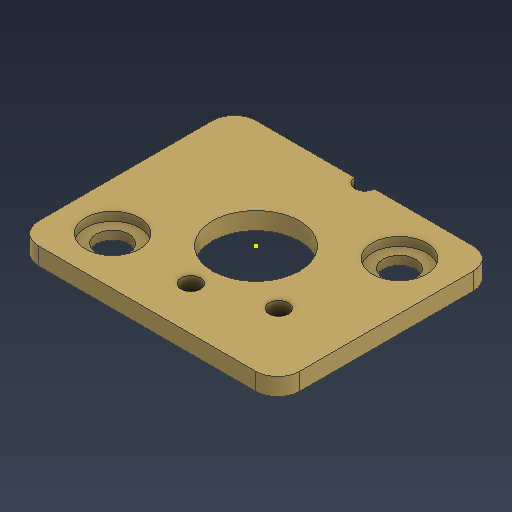
# Autodesk Inventor part: Chapa Inferior
Saved by Autodesk Inventor 2021 (Build 250183000, 183)
## iProperties
Created: 2021-01-18
Part Number: Chapa Inferior
Material: Genérico
Document SubType Name: Modeling
Designer: João
Density: 1 g/cm^3
Appearance: Padrão
Author: João
Autodesk Inventor part; units mm, degrees
ref_plane "YZ Plane" through (0, 0, 0) normal (1, 0, 0) x (0, 1, 0)
ref_plane "XZ Plane" through (0, 0, 0) normal (0, 1, 0) x (-1, 0, 0)
ref_plane "XY Plane" through (0, 0, 0) normal (0, 0, 1) x (1, 0, 0)
sketch "Esboço2" plane through (0, 0, 0) normal (0, 1, 0) x (-1, 0, 0)
  circle A0 centre (3.8014, 2.7994) radius 1.25
  circle A1 centre (-3.8014, -2.7994) radius 1.25
  arc A2 (-5, 5) -> (-6, 4) centre (-5, 4) ccw
  line L0 (-6, 4) -> (-6, -4)
  arc A3 (-6, -4) -> (-5, -5) centre (-5, -4) ccw
  line L1 (-5, -5) -> (5, -5)
  arc A4 (5, -5) -> (6, -4) centre (5, -4) ccw
  line L2 (6, -4) -> (6, 4)
  arc A5 (6, 4) -> (5, 5) centre (5, 4) ccw
  line L3 (5, 5) -> (-5, 5)
  circle A6 centre (0, 0) radius 2
  arc A7 (0.45, -5) -> (-0.45, -5) centre (0, -5) ccw
  circle A8 centre (3.8014, 2.7994) radius 0.75
  circle A9 centre (-3.8014, -2.7994) radius 0.75
  circle A10 centre (-3.0146, 1.9633) radius 0.45
  circle A11 centre (0, 3) radius 0.45
  line L4 (0, 0) -> (0, 5)
  dimension "d16" = 0.9
  dimension "d17" = 1.5
  dimension "d18" = 1.5
  dimension "d23" = 4
  dimension "d26" = 2
  dimension "d27" = 0
  constraints: 12 centre point, 10 end point, 10 point on circle, 2 coincident, 2 midpoint, 2 point on line
  measures "d16" diameter of A7
  measures "d17" diameter of A8
  measures "d18" diameter of A9
  measures "d23" diameter of A6
  measures "d26" distance from line of L3 A11.centre
  measures "d27" distance from line of L4 A11.centre
extrude "Extrusão3" add sketch "Esboço2" along normal blind 0.8 contours A11 L4 | L4 A11 | L3 A5 L2 A4 L1 A7 A3 L0 A2 | A10
extrude "Extrusão4" add sketch "Esboço2" along normal blind 0.4 contours A0 | A1
extrude "Extrusão5" cut sketch "Esboço2" along normal blind 10 contours A10
extrude "Extrusão6" cut sketch "Esboço2" along normal blind 10 contours A11 L4 | L4 A11
sketch "Esboço4" plane through (0, 0.8, 0) normal (0, 1, 0) x (1, 0, 0)
  point P0 (0, 0)
